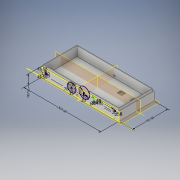
# Autodesk Inventor part: 0811_bottom
Saved by Autodesk Inventor 2019 (Build 230136000, 136)
## iProperties
Created: 2019-08-11
Part Number: 0811_bottom
Material: Generic
Document SubType Name: Modeling
Designer: tmst0
Density: 1 g/cm^3
Appearance: Default
Author: tmst0
Autodesk Inventor part; units mm, degrees
sketch "Sketch3" plane through (0, 0, 0) normal (0, 1, 0) x (-1, 0, 0)
  line L0 (101.5, -46.5) -> (-101.5, -46.5)
  line L1 (-101.5, -46.5) -> (-101.5, 46.5)
  line L2 (-101.5, 46.5) -> (101.5, 46.5)
  line L3 (101.5, 46.5) -> (101.5, -46.5)
  line L4 (101.5, -46.5) -> (-101.5, 46.5) construction
  line L5 (-101.5, -46.5) -> (101.5, 46.5) construction
  point P0 (0, 0)
  dimension "d13" = 203
  dimension "d14" = 93
  constraints: 12 end point, 2 midpoint, 2 parallel, 1 horizontal, 1 perpendicular
  measures "d13" distance of L0.start L0.end
  measures "d14" distance of L2.end L0.start
extrude "Extrusion3" add sketch "Sketch3" along normal blind 28
shell "Shell2" thickness 3 removed faces 1 at (33.8333, 28, -15.5)
sketch "Sketch7" plane through (0, 0, 0) normal (0, 1, 0) x (-1, 0, 0)
  line L0 (100, -45) -> (-100, -45)
  line L1 (-100, -45) -> (-100, 45)
  line L2 (-100, 45) -> (100, 45)
  line L3 (100, 45) -> (100, -45)
  line L4 (100, -45) -> (-100, 45) construction
  line L5 (-100, -45) -> (100, 45) construction
  line L6 (102.5, -47.5) -> (-102.5, -47.5)
  line L7 (-102.5, -47.5) -> (-102.5, 47.5)
  line L8 (-102.5, 47.5) -> (102.5, 47.5)
  line L9 (102.5, 47.5) -> (102.5, -47.5)
  line L10 (102.5, -47.5) -> (-102.5, 47.5) construction
  line L11 (-102.5, -47.5) -> (102.5, 47.5) construction
  point P0 (0, 0)
  dimension "d31" = 200
  dimension "d32" = 90
  dimension "d33" = 205
  dimension "d34" = 95
  constraints: 24 end point, 4 midpoint, 4 parallel, 2 horizontal, 2 perpendicular
  measures "d31" distance of L1.end L2.end
  measures "d32" distance of L0.end L1.end
  measures "d33" distance of L7.end L8.end
  measures "d34" distance of L6.end L7.end
extrude "Extrusion6" add sketch "Sketch7" along normal blind 5 separate body
move or copy body "Move Body2" bodies to move or copy 2 copy no translate (0, 23, 0)
combine bodies "Combine1" operation type subtract main body 1 bodies to subtract 2
sketch "Sketch10" plane through (-101.5, 0, 46.5) normal (0, 0, 1) x (1, 0, 0)
  circle A0 centre (192.5, 20) radius 2.4
  line L0 (203, 0) -> (0, 0) projected
  line L1 (203, 0) -> (203, 23) projected
  circle A1 centre (137.5, 19) radius 2.4
  circle A2 centre (111.5, 20) radius 14
  line L2 (7.4, 14.4798) -> (15.4, 14.4798)
  line L3 (15.4, 14.4798) -> (15.4, 12.4798)
  line L4 (7.4, 12.4798) -> (7.4, 14.4798)
  line L5 (7.4, 12.4798) -> (8.4, 11.5)
  line L6 (8.4, 11.5) -> (14.4, 11.5)
  line L7 (14.4, 11.5) -> (15.4, 12.4798)
  line L8 (0, 0) -> (0, 23) projected
  point P0 (101.5, 0)
  dimension "d42" = 4.8
  dimension "d43" = 20
  dimension "d44" = 10.5
  dimension "d45" = 4.8
  dimension "d46" = 55
  dimension "d47" = 28
  dimension "d48" = 20
  dimension "d49" = 91.5
  dimension "d50" = 8
  dimension "d51" = 2
  dimension "d54" = 1.4
  dimension "d55" = 6
  dimension "d56" = 7.4
  dimension "d57" = 11.5
  dimension "d58" = 45.585
  dimension "d59" = 45.585
  constraints: 12 end point, 3 centre point, 2 horizontal, 1 perpendicular
  measures "d42" diameter of A0
  measures "d43" distance from line of L0 A0.centre
  measures "d44" distance from line of L1 A0.centre
  measures "d45" diameter of A1
  measures "d46" horizontal distance of A1.centre A0.centre
  measures "d47" diameter of A2
  measures "d48" distance from line of L0 A2.centre
  measures "d49" distance from line of L1 A2.centre
  measures "d50" distance of L2.start L2.end
  measures "d51" distance of L2.end L3.end
  measures "d54" distance of L4.start L5.end
  measures "d55" distance of L5.end L6.end
  measures "d56" distance between parallel lines of L8 L4
  measures "d57" distance between parallel lines of L0 L6
  measures "d58" angle of L8 L5
  measures "d59" angle of L8 L7
sketch "Sketch11" plane through (0, 0, 0) normal (0, 0, 1) x (1, 0, 0)
  point P0 (0, 0)
sketch "Sketch12" plane through (-101.5, 0, 46.5) normal (0, 0, 1) x (1, 0, 0)
  circle A0 centre (78.5, 15) radius 11.5
  line L0 (0, 0) -> (0, 23) projected
  line L1 (-40.6, 0) -> (243.6, 0) projected
  line L2 (203, 23) -> (0, 23) projected
  line L3 (203, 0) -> (203, 23) projected
  point P0 (101.5, 0)
  dimension "d60" = 23
  dimension "d61" = 78.5
  dimension "d62" = 15
  dimension "d92" = 8
  dimension "d93" = 124.5
  constraints: 1 centre point
  measures "d60" diameter of A0
  measures "d61" distance from line of L0 A0.centre
  measures "d62" distance from line of L1 A0.centre
  measures "d92" distance from line of L2 A0.centre
  measures "d93" distance from line of L3 A0.centre
sketch "Sketch13" plane through (101.5, 0, -46.5) normal (0, 0, -1) x (-1, 0, 0)
  circle A0 centre (6, 18) radius 2.7
  line L0 (0, 0) -> (0, 23) projected
  line L1 (1.5, 28) -> (201.5, 28) projected
  circle A1 centre (101.5, 8.5) radius 2.4
  line L2 (203, 0) -> (0, 0) projected
  point P0 (101.5, 0)
  dimension "d63" = 5.4
  dimension "d64" = 6
  dimension "d65" = 10
  dimension "d66" = 4.8
  dimension "d67" = 8.5
  constraints: 2 centre point
  measures "d63" diameter of A0
  measures "d64" distance from line of L0 A0.centre
  measures "d65" distance from line of L1 A0.centre
  measures "d66" diameter of A1
  measures "d67" distance from line of L2 A1.centre
sketch "Sketch14" plane through (-101.5, 0, 46.5) normal (0, 0, 1) x (1, 0, 0)
  circle A0 centre (94, 5.4) radius 2.4
  line L0 (-40.6, 0) -> (243.6, 0) projected
  point P0 (101.5, 0)
  dimension "d68" = 4.8
  dimension "d69" = 5.4
  constraints: 1 centre point
  measures "d68" diameter of A0
  measures "d69" distance from line of L0 A0.centre
sketch "Sketch15" plane through (-98.5, 3, -43.5) normal (0, 1, 0) x (1, 0, 0)
  line L0 (171.5, -20) -> (181, -20)
  line L1 (182.5, -21.5) -> (182.5, -28.5)
  line L2 (181, -30) -> (171.5, -30)
  line L3 (170, -28.5) -> (170, -21.5)
  line L4 (170, -20) -> (182.5, -30) construction
  line L5 (182.5, -20) -> (170, -30) construction
  arc A0 (171.5, -20) -> (170, -21.5) centre (171.5, -21.5) ccw
  arc A1 (170, -28.5) -> (171.5, -30) centre (171.5, -28.5) ccw
  arc A2 (182.5, -21.5) -> (181, -20) centre (181, -21.5) ccw
  arc A3 (181, -30) -> (182.5, -28.5) centre (181, -28.5) ccw
  line L6 (137, -20) -> (146.5, -20)
  line L7 (148, -21.5) -> (148, -28.5)
  line L8 (146.5, -30) -> (137, -30)
  line L9 (135.5, -28.5) -> (135.5, -21.5)
  line L10 (135.5, -20) -> (148, -30) construction
  line L11 (148, -20) -> (135.5, -30) construction
  arc A4 (137, -20) -> (135.5, -21.5) centre (137, -21.5) ccw
  arc A5 (135.5, -28.5) -> (137, -30) centre (137, -28.5) ccw
  arc A6 (148, -21.5) -> (146.5, -20) centre (146.5, -21.5) ccw
  arc A7 (146.5, -30) -> (148, -28.5) centre (146.5, -28.5) ccw
  line L12 (197, 0) -> (197, -87) projected
  line L13 (0, 0) -> (197, 0) projected
  point P0 (98.5, -43.5)
  point P1 (176.25, -25)
  point P2 (141.75, -25)
  dimension "d70" = 12.5
  dimension "d71" = 10
  dimension "d72" = 1.5
  dimension "d73" = 12.5
  dimension "d74" = 10
  dimension "d75" = 1.5
  dimension "d76" = 14.5
  dimension "d77" = 22
  dimension "d78" = 20
  dimension "d79" = 20
  constraints: 24 end point, 16 point on circle, 16 point on line, 16 tangent, 8 centre point, 6 equal radius, 4 midpoint, 4 parallel, 2 horizontal, 2 perpendicular
  measures "d70" distance of L4.start L5.start
  measures "d71" distance of L5.start L4.end
  measures "d72" radius of A0
  measures "d73" distance of L10.start L11.start
  measures "d74" distance of L11.start L10.end
  measures "d75" radius of A4
  measures "d76" distance between parallel lines of L12 L1
  measures "d77" distance between parallel lines of L7 L3
  measures "d78" distance between parallel lines of L13 L0
  measures "d79" distance between parallel lines of L13 L6
extrude "Extrusion7" cut sketch "Sketch15" against normal blind 62.75 bodies 1
extrude "Extrusion8" cut sketch "Sketch10" against normal blind 4.8 contours A0 | A1 | L2 L3 L7 L6 L5 L4 bodies 1
extrude "Extrusion9" cut sketch "Sketch14" against normal blind 4.8 bodies 1
extrude "Extrusion10" cut sketch "Sketch13" against normal blind 4.8 bodies 1
extrude "Extrusion11" add sketch "Sketch12" along normal mid plane 50 separate body contours A0 L2 | L2 A0
extrude "Extrusion12" add sketch "Sketch10" along normal mid plane 50 separate body contours A2
combine bodies "Combine2" operation type subtract main body 1 bodies to subtract 3 4
equation "\"d82\" = d68"
equation "\"d84\" = d68"
equation "\"d86\" = d68"
body "Solid2"
